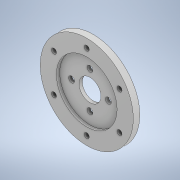
# Autodesk Inventor part: Leg_joint_cross_bearing_frame
Saved by Autodesk Inventor 2020.4 (Build 244396000, 396)
## iProperties
Created: 2021-09-21
Part Number: Leg_joint_cross_bearing_frame
Material: アルミニウム 2014-T4
Document SubType Name: Modeling
Designer: Masato
Density: 2.8 g/cm^3
Appearance: 滑らか - 淡い灰色
Author: Masato
Autodesk Inventor part; units mm, degrees
ref_plane "YZ Plane" through (0, 0, 0) normal (1, 0, 0) x (0, 1, 0)
ref_plane "XZ Plane" through (0, 0, 0) normal (0, 1, 0) x (-1, 0, 0)
ref_plane "XY Plane" through (0, 0, 0) normal (0, 0, 1) x (1, 0, 0)
sketch "スケッチ1" plane through (0, 0, 0) normal (0, 0, 1) x (1, 0, 0)
  circle A0 centre (0, 0) radius 21.5
  circle A1 centre (0, 0) radius 14
  line L0 (0, 21.5) -> (0, -21.5) construction
  circle A2 centre (0, 17.5) radius 1.15
  circle A3 centre (-15.1554, 8.75) radius 1.15
  circle A4 centre (-15.1554, -8.75) radius 1.15
  circle A5 centre (0, -17.5) radius 1.15
  circle A6 centre (15.1554, -8.75) radius 1.15
  circle A7 centre (15.1554, 8.75) radius 1.15
  circle A8 centre (0, 8.5) radius 1.35
  circle A9 centre (-8.5, 0) radius 1.35
  circle A10 centre (0, -8.5) radius 1.35
  circle A11 centre (8.5, 0) radius 1.35
  circle A12 centre (0, 0) radius 5.05
  dimension "d0" = 43
  dimension "d1" = 28
  dimension "d2" = 2.3
  dimension "d3" = 17.5
  dimension "d6" = 360
  dimension "d8" = 2.7
  dimension "d9" = 8.5
  dimension "d12" = 360
  dimension "d16" = 10.1
  constraints: 13 centre point, 5 coincident, 2 end point, 2 point on circle, 2 point on line, 1 midpoint, 1 vertical, 24 other
  measures "d0" diameter of A0
  measures "d1" diameter of A1
  measures "d2" diameter of A2
  measures "d3" distance of point (0, 0) A2.centre
  measures "d8" diameter of A8
  measures "d9" distance of point (0, 0) A8.centre
  measures "d16" diameter of A12
extrude "押し出し1" add sketch "スケッチ1" along normal blind 3 contours A0
extrude "押し出し2" add sketch "スケッチ1" along normal blind 1.5 contours A1
